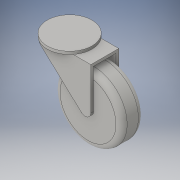
# Autodesk Inventor part: Caster Placeholder
Saved by Autodesk Inventor 2016 (Build 200138000, 138)
## iProperties
Created: 2017-11-04
Part Number: Caster Placeholder
Material: Wood (Oak)
Document SubType Name: Modeling
Designer: mathaetaes
Density: 0.76 g/cm^3
Appearance: White Oak - Natural Medium Gloss
Author: mathaetaes
Autodesk Inventor part; units mm, degrees
ref_plane "YZ Plane" through (0, 0, 0) normal (1, 0, 0) x (0, 1, 0)
ref_plane "XZ Plane" through (0, 0, 0) normal (0, 1, 0) x (-1, 0, 0)
ref_plane "XY Plane" through (0, 0, 0) normal (0, 0, 1) x (1, 0, 0)
sketch "Sketch1" plane through (0, 0, 0) normal (0, 0, 1) x (1, 0, 0)
  circle A0 centre (0, 0) radius 38.1
  dimension "d0" = 76.2
  constraints: 1 centre point, 1 coincident
  measures "d0" diameter of A0
extrude "Extrusion1" add sketch "Sketch1" along normal blind 25.4
fillet "Fillet1" radius 6.35 2 edges at (-38.1, 0, 25.4) (-38.1, 0, 0)
sketch "Sketch3" plane through (0, 0, 25.4) normal (0, 0, 1) x (1, 0, 0)
  line L0 (6.35, 44.45) -> (-53.2838, 44.45)
  circle A0 centre (0, 0) radius 38.1 projected
  arc A1 (-4.3231, -4.6511) -> (6.35, 0) centre (0, 0) ccw
  line L1 (6.35, 0) -> (6.35, 44.45)
  arc A2 (-53.2838, 44.45) -> (-47.6982, 35.6648) centre (-39.6513, 46.9493) ccw
  line L2 (-50.3182, 38.1) -> (-4.3231, -4.6511)
  dimension "d8" = 44.45
  dimension "d9" = 76.2
  dimension "d10" = 12.7
  constraints: 7 end point, 5 point on circle, 2 centre point, 2 tangent, 1 coincident, 1 horizontal, 1 perpendicular, 1 point on line
  measures "d8" distance from line of A0.centre L0
  measures "d9" diameter of A0
  measures "d10" diameter of A1
extrude "Extrusion2" add sketch "Sketch3" along normal blind 3.175 contours L1 A0 L2 A2 L0 | L1 A1 L2 A0 picked at (-4.398, 10.0922)
pattern_linear "Rectangular Pattern1" count 2 spacing 28.575 along (0, 0, -1) of "Extrusion2"
sketch "Sketch4" plane through (-53.2838, 44.45, 25.4) normal (0, 1, 0) x (1, 0, 0)
  line L0 (59.6338, -3.175) -> (0, -3.175) projected
  line L1 (59.6338, 28.575) -> (0, 28.575) projected
  line L2 (0, -3.175) -> (59.6338, -3.175)
  line L3 (59.6338, -3.175) -> (59.6338, 28.575)
  line L4 (59.6338, 28.575) -> (0, 28.575)
  line L5 (0, 28.575) -> (0, -3.175)
  point P0 (53.2838, 25.4)
  dimension "d20" = 31.75
  constraints: 8 end point, 2 parallel, 1 horizontal, 1 perpendicular
  measures "d20" distance of L4.end L0.end
extrude "Extrusion3" add sketch "Sketch4" along normal blind 3.175
sketch "Sketch5" plane through (-53.2838, 47.625, 25.4) normal (0, 1, 0) x (1, 0, 0)
  circle A0 centre (19.7076, 12.7) radius 25.4
  line L0 (59.6338, 28.575) -> (0, 28.575) projected
  line L1 (59.6338, -3.175) -> (59.6338, 28.575) projected
  dimension "d19" = 15.875
  dimension "d21" = 50.8
  constraints: 1 centre point
  measures "d19" distance from line of L0 A0.centre
  measures "d21" diameter of A0
extrude "Extrusion4" add sketch "Sketch5" along normal blind 3.175
equation "\"d19\" = 0.5 * d20"
body "Solid1"
